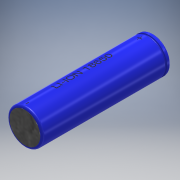
# Autodesk Inventor part: Bateria 18650
Saved by Autodesk Inventor 2018 (Build 220112000, 112)
## iProperties
Created: 2017-09-13
Part Number: Bateria 18650
Material: Genérico
Document SubType Name: Modeling
Designer: Julio Orozco
Density: 1 g/cm^3
Appearance: Valor por defecto
Author: Julio Orozco
Autodesk Inventor part; units mm, degrees
note: some values were not read from the file. Chosen so that the rebuilt part matches the saved one: direction of "Repujado1".
ref_plane "YZ Plane" through (0, 0, 0) normal (1, 0, 0) x (0, 1, 0)
sketch "Boceto1" plane through (0, 0, 0) normal (0, 1, 0) x (-1, 0, 0)
  circle A0 centre (0, 0) radius 9
  dimension "d0" = 18
  constraints: 1 centre point, 1 coincident
  measures "d0" diameter of A0
extrude "Extrusión1" add sketch "Boceto1" along normal blind 65
sketch "Boceto2" plane through (0, 0, 0) normal (0, 0, 1) x (1, 0, 0)
  line L0 (0, 0) -> (0, 65) construction
  line L1 (9, 65) -> (-9, 65) projected
  line L2 (9, 0) -> (9, 65) projected
  circle A0 centre (9, 62.5) radius 0.5
  dimension "d3" = 1
  dimension "d4" = 2.5
  constraints: 2 end point, 1 centre point, 1 midpoint, 1 point on line
  measures "d3" diameter of A0
  measures "d4" distance from line of A0.centre L1
revolve "Revolución1" cut sketch "Boceto2" angle 360 about axis through (0, 0, 0) along (0, 1, 0)
fillet "Empalme1" radius 1 2 edges at (9, 65, 0) (9, 0, 0)
ref_plane "Plano de trabajo1" through (0, 66, 0) normal (0, 1, 0) x (1, 0, 0)
sketch "Boceto3" plane through (0, 66, 0) normal (0, 1, 0) x (1, 0, 0)
  circle A0 centre (0, 0) radius 3.5
  dimension "d8" = 7
  constraints: 1 centre point, 1 coincident
  measures "d8" diameter of A0
extrude "Extrusión2" add sketch "Boceto3" against normal blind 0.1
sketch "Boceto4" plane through (0, 0, 0) normal (0, 0, 1) x (1, 0, 0)
  line L0 (-8, 65) -> (8, 65) projected
  line L1 (-3.5, 66) -> (3.5, 66) projected
  arc A0 (8, 65) -> (3.5, 66) centre (3.5, 55.375) ccw
  arc A1 (7.7585, 65) -> (3.5, 65.9) centre (3.5, 55.375) ccw
  line L2 (-3.5, 65.9) -> (3.5, 65.9) projected
  line L3 (3.5, 65.9) -> (3.5, 66)
  line L4 (7.7585, 65) -> (8, 65)
  line L5 (0, 65.9) -> (0, 63.9288) construction
  point P0 (0, 0)
  dimension "d11" = 0.1
  constraints: 6 end point, 4 point on circle, 2 centre point, 1 collinear, 1 midpoint, 1 perpendicular, 1 point on line, 1 tangent, 1 vertical
  measures "d11" radial gap between concentric circles of A0 A1
revolve "Revolución2" add sketch "Boceto4" angle 360 about axis through (0, 65.9, 0) along (0, -1, 0)
sketch "Boceto5" plane through (0, 66, 0) normal (0, 1, 0) x (1, 0, 0)
  line L0 (-6.8, -1.2007) -> (-6.8, 1.2993) construction
  line L1 (-5.6, -1.2007) -> (-5.6, 1.2993)
  line L2 (-8, 1.2993) -> (-8, -1.2007)
  arc A0 (-8, -1.2007) -> (-5.6, -1.2007) centre (-6.8, -1.2007) ccw
  arc A1 (-5.6, 1.2993) -> (-8, 1.2993) centre (-6.8, 1.2993) ccw
  point P0 (0, 0)
  point P1 (-6.8, 0.0493)
  dimension "d13" = 1.2
  dimension "d14" = 2.5
  dimension "d15" = 6.8
  constraints: 8 end point, 4 point on circle, 4 tangent, 2 centre point, 1 midpoint, 1 parallel, 1 vertical
  measures "d13" radius of A1
  measures "d14" distance of L1.start L1.end
  measures "d15" horizontal distance of point (0, 0) point (-6.8, 0.049)
extrude "Extrusión4" cut sketch "Boceto5" against normal blind 1
pattern_circular "Patrón circular1" count 6 over 360 about axis through (0, 0, 0) along (0, 1, 0) of "Extrusión4"
sketch "Boceto6" plane through (0, 0, 0) normal (0, -1, 0) x (1, 0, 0)
  circle A0 centre (0, 0) radius 7.7585
  constraints: 1 centre point, 1 coincident
extrude "Extrusión5" add sketch "Boceto6" along normal blind 0.1
ref_plane "Plano de trabajo2" through (0, 0, 9) normal (0, 0, 1) x (1, 0, 0)
sketch "Boceto7" plane through (0, 0, 9) normal (0, 0, 1) x (1, 0, 0)
  line L0 (-3.1701, 1.4356) -> (-3.1701, 76.7108) construction
  line L1 (-3.1701, 76.7108) -> (-0.0107, 76.7108) construction
  line L2 (-0.0107, 76.7108) -> (-0.0107, 1.4356) construction
  line L3 (-0.0107, 1.4356) -> (-3.1701, 1.4356) construction
  line L4 (-1.0179, 1.6337) -> (-1.3827, 1.6337)
  line L5 (-1.3827, 1.6337) -> (-1.3827, 3.1602)
  line L6 (-1.3827, 3.1602) -> (-1.0179, 3.1602)
  line L7 (-1.0179, 3.1602) -> (-1.0179, 1.6337)
  line L8 (-0.0904, 16.1602) -> (-3.0904, 16.1602)
  line L9 (-3.0904, 16.1602) -> (-3.0904, 16.5853)
  line L10 (-3.0904, 16.5853) -> (-0.4938, 16.5853)
  line L11 (-0.4938, 16.5853) -> (-0.4938, 18.4211)
  line L12 (-0.4938, 18.4211) -> (-0.0904, 18.4211)
  line L13 (-0.0904, 18.4211) -> (-0.0904, 16.1602)
  line L14 (-0.0904, 18.8535) -> (-3.0904, 18.8535)
  line L15 (-3.0904, 18.8535) -> (-3.0904, 19.2786)
  line L16 (-3.0904, 19.2786) -> (-0.0904, 19.2786)
  line L17 (-0.0904, 19.2786) -> (-0.0904, 18.8535)
  line L18 (-1.0179, 19.8486) -> (-1.3827, 19.8486)
  line L19 (-1.3827, 19.8486) -> (-1.3827, 21.3752)
  line L20 (-1.3827, 21.3752) -> (-1.0179, 21.3752)
  line L21 (-1.0179, 21.3752) -> (-1.0179, 19.8486)
  line L22 (-0.0904, 21.9477) -> (-3.0904, 21.9477)
  line L23 (-3.0904, 21.9477) -> (-3.0904, 22.3728)
  line L24 (-3.0904, 22.3728) -> (-0.0904, 22.3728)
  line L25 (-0.0904, 22.3728) -> (-0.0904, 21.9477)
  spline S0 degree 2 poles (-1.5904, 22.9235) (-2.315, 22.9235) (-3.1701, 23.81) (-3.1701, 24.5684) knots 0 0 0 1 2 2 2
  spline S1 degree 2 poles (-3.1701, 24.5684) (-3.1701, 25.3269) (-2.315, 26.211) (-1.5904, 26.211) knots 0 0 0 1 2 2 2
  spline S2 degree 2 poles (-1.5904, 26.211) (-0.8634, 26.211) (-0.0107, 25.3245) (-0.0107, 24.566) knots 0 0 0 1 2 2 2
  spline S3 degree 2 poles (-0.0107, 24.566) (-0.0107, 23.8076) (-0.8634, 22.9235) (-1.5904, 22.9235) knots 0 0 0 1 2 2 2
  spline S4 degree 2 poles (-1.5904, 23.3631) (-1.0324, 23.3631) (-0.4093, 24.0008) (-0.4093, 24.5684) knots 0 0 0 1 2 2 2
  spline S5 degree 2 poles (-0.4093, 24.5684) (-0.4093, 25.1361) (-1.0349, 25.7713) (-1.5904, 25.7713) knots 0 0 0 1 2 2 2
  spline S6 degree 2 poles (-1.5904, 25.7713) (-2.146, 25.7713) (-2.7716, 25.1337) (-2.7716, 24.566) knots 0 0 0 1 2 2 2
  spline S7 degree 2 poles (-2.7716, 24.566) (-2.7716, 23.9984) (-2.146, 23.3631) (-1.5904, 23.3631) knots 0 0 0 1 2 2 2
  line L26 (-0.0904, 26.7327) -> (-3.0904, 26.7327)
  line L27 (-3.0904, 26.7327) -> (-3.0904, 27.3076)
  line L28 (-3.0904, 27.3076) -> (-0.53, 29.1965)
  line L29 (-0.53, 29.1965) -> (-3.0904, 29.1965)
  line L30 (-3.0904, 29.1965) -> (-3.0904, 29.6071)
  line L31 (-3.0904, 29.6071) -> (-0.0904, 29.6071)
  line L32 (-0.0904, 29.6071) -> (-0.0904, 29.0346)
  line L33 (-0.0904, 29.0346) -> (-2.6508, 27.1481)
  line L34 (-2.6508, 27.1481) -> (-0.0904, 27.1481)
  line L35 (-0.0904, 27.1481) -> (-0.0904, 26.7327)
  line L36 (-0.0904, 32.6385) -> (-2.1991, 32.6385)
  line L37 (-2.1991, 32.6385) -> (-2.1991, 31.7448)
  line L38 (-2.1991, 31.7448) -> (-2.5445, 31.7448)
  line L39 (-2.5445, 31.7448) -> (-2.5445, 31.81)
  spline S8 degree 2 poles (-2.5445, 31.81) (-2.5445, 32.2617) (-2.8054, 32.7013) (-3.0904, 32.7303) knots 0 0 0 1 2 2 2
  line L40 (-3.0904, 32.7303) -> (-3.0904, 33.0467)
  line L41 (-3.0904, 33.0467) -> (-0.0904, 33.0467)
  line L42 (-0.0904, 33.0467) -> (-0.0904, 32.6385)
  spline S9 degree 2 poles (-1.6991, 34.9573) (-1.7643, 34.694) (-2.0759, 34.4163) (-2.3006, 34.4163) knots 0 0 0 1 2 2 2
  spline S10 degree 2 poles (-2.3006, 34.4163) (-2.6653, 34.4163) (-3.0904, 35.0081) (-3.0904, 35.525) knots 0 0 0 1 2 2 2
  spline S11 degree 2 poles (-3.0904, 35.525) (-3.0904, 36.0032) (-2.658, 36.5781) (-2.3006, 36.5781) knots 0 0 0 1 2 2 2
  spline S12 degree 2 poles (-2.3006, 36.5781) (-2.0759, 36.5781) (-1.7643, 36.2979) (-1.6991, 36.037) knots 0 0 0 1 2 2 2
  spline S13 degree 2 poles (-1.6991, 36.037) (-1.6291, 36.3655) (-1.2474, 36.694) (-0.9382, 36.694) knots 0 0 0 1 2 2 2
  spline S14 degree 2 poles (-0.9382, 36.694) (-0.5059, 36.694) (-0.0107, 36.0564) (-0.0107, 35.496) knots 0 0 0 1 2 2 2
  spline S15 degree 2 poles (-0.0107, 35.496) (-0.0107, 34.9404) (-0.5107, 34.2955) (-0.9382, 34.2955) knots 0 0 0 1 2 2 2
  spline S16 degree 2 poles (-0.9382, 34.2955) (-1.245, 34.2955) (-1.6411, 34.6385) (-1.6991, 34.9573) knots 0 0 0 1 2 2 2
  spline S17 degree 2 poles (-0.9745, 36.2544) (-1.2281, 36.2544) (-1.5131, 35.851) (-1.5131, 35.4887) knots 0 0 0 1 2 2 2
  spline S18 degree 2 poles (-1.5131, 35.4887) (-1.5131, 35.1216) (-1.2305, 34.7206) (-0.9745, 34.7206) knots 0 0 0 1 2 2 2
  spline S19 degree 2 poles (-0.9745, 34.7206) (-0.7112, 34.7206) (-0.402, 35.1288) (-0.402, 35.4767) knots 0 0 0 1 2 2 2
  spline S20 degree 2 poles (-0.402, 35.4767) (-0.402, 35.8438) (-0.7039, 36.2544) (-0.9745, 36.2544) knots 0 0 0 1 2 2 2
  spline S21 degree 2 poles (-2.3006, 36.1361) (-2.5059, 36.1361) (-2.7329, 35.8076) (-2.7329, 35.5081) knots 0 0 0 1 2 2 2
  spline S22 degree 2 poles (-2.7329, 35.5081) (-2.7329, 35.1892) (-2.5107, 34.8535) (-2.3006, 34.8535) knots 0 0 0 1 2 2 2
  spline S23 degree 2 poles (-2.3006, 34.8535) (-2.0928, 34.8535) (-1.8465, 35.1989) (-1.8465, 35.496) knots 0 0 0 1 2 2 2
  spline S24 degree 2 poles (-1.8465, 35.496) (-1.8465, 35.7931) (-2.0928, 36.1361) (-2.3006, 36.1361) knots 0 0 0 1 2 2 2
  spline S25 degree 2 poles (-1.5735, 37.496) (-1.8054, 37.6699) (-2.03, 38.1482) (-2.03, 38.4549) knots 0 0 0 1 2 2 2
  spline S26 degree 2 poles (-2.03, 38.4549) (-2.03, 38.9283) (-1.4938, 39.5105) (-1.0614, 39.5105) knots 0 0 0 1 2 2 2
  spline S27 degree 2 poles (-1.0614, 39.5105) (-0.5952, 39.5105) (-0.0107, 38.8317) (-0.0107, 38.2858) knots 0 0 0 1 2 2 2
  spline S28 degree 2 poles (-0.0107, 38.2858) (-0.0107, 37.6892) (-0.7667, 37.0467) (-1.4696, 37.0467) knots 0 0 0 1 2 2 2
  spline S29 degree 2 poles (-1.4696, 37.0467) (-2.2522, 37.0467) (-3.0952, 37.7254) (-3.0952, 38.3559) knots 0 0 0 1 2 2 2
  spline S30 degree 2 poles (-3.0952, 38.3559) (-3.0952, 38.7834) (-2.7088, 39.3196) (-2.3585, 39.3776) knots 0 0 0 1 2 2 2
  line L43 (-2.3585, 39.3776) -> (-2.3585, 38.9525)
  spline S31 degree 2 poles (-2.3585, 38.9525) (-2.5421, 38.8945) (-2.7329, 38.5902) (-2.7329, 38.3559) knots 0 0 0 1 2 2 2
  spline S32 degree 2 poles (-2.7329, 38.3559) (-2.7329, 37.9259) (-2.1532, 37.496) (-1.5735, 37.496) knots 0 0 0 1 2 2 2
  spline S33 degree 2 poles (-1.0276, 37.5515) (-0.7498, 37.5515) (-0.4093, 37.9597) (-0.4093, 38.2931) knots 0 0 0 1 2 2 2
  spline S34 degree 2 poles (-0.4093, 38.2931) (-0.4093, 38.653) (-0.7547, 39.0829) (-1.0373, 39.0829) knots 0 0 0 1 2 2 2
  spline S35 degree 2 poles (-1.0373, 39.0829) (-1.3223, 39.0829) (-1.6725, 38.6602) (-1.6725, 38.3148) knots 0 0 0 1 2 2 2
  spline S36 degree 2 poles (-1.6725, 38.3148) (-1.6725, 37.9791) (-1.3102, 37.5515) (-1.0276, 37.5515) knots 0 0 0 1 2 2 2
  line L44 (-0.8948, 39.8414) -> (-0.8948, 40.2689)
  spline S37 degree 2 poles (-0.8948, 40.2689) (-0.6484, 40.31) (-0.3972, 40.6651) (-0.3972, 40.9718) knots 0 0 0 1 2 2 2
  spline S38 degree 2 poles (-0.3972, 40.9718) (-0.3972, 41.3269) (-0.7716, 41.7641) (-1.0687, 41.7641) knots 0 0 0 1 2 2 2
  spline S39 degree 2 poles (-1.0687, 41.7641) (-1.3634, 41.7641) (-1.7281, 41.3366) (-1.7281, 40.9936) knots 0 0 0 1 2 2 2
  spline S40 degree 2 poles (-1.7281, 40.9936) (-1.7281, 40.7689) (-1.5687, 40.4332) (-1.4117, 40.3366) knots 0 0 0 1 2 2 2
  line L45 (-1.4117, 40.3366) -> (-1.4117, 39.9211)
  line L46 (-1.4117, 39.9211) -> (-3.0155, 40.182)
  line L47 (-3.0155, 40.182) -> (-3.0155, 41.9815)
  line L48 (-3.0155, 41.9815) -> (-2.6363, 41.9815)
  line L49 (-2.6363, 41.9815) -> (-2.6363, 40.5032)
  line L50 (-2.6363, 40.5032) -> (-1.8102, 40.3607)
  spline S41 degree 2 poles (-1.8102, 40.3607) (-1.9431, 40.4936) (-2.0759, 40.868) (-2.0759, 41.1095) knots 0 0 0 1 2 2 2
  spline S42 degree 2 poles (-2.0759, 41.1095) (-2.0759, 41.3003) (-1.989, 41.6312) (-1.902, 41.7641) knots 0 0 0 1 2 2 2
  spline S43 degree 2 poles (-1.902, 41.7641) (-1.7667, 41.9718) (-1.3465, 42.2061) (-1.1001, 42.2061) knots 0 0 0 1 2 2 2
  spline S44 degree 2 poles (-1.1001, 42.2061) (-0.6146, 42.2061) (-0.0107, 41.5274) (-0.0107, 40.9742) knots 0 0 0 1 2 2 2
  spline S45 degree 2 poles (-0.0107, 40.9742) (-0.0107, 40.4887) (-0.4793, 39.8873) (-0.8948, 39.8414) knots 0 0 0 1 2 2 2
  spline S46 degree 2 poles (-1.5518, 42.6047) (-2.2909, 42.6047) (-3.0904, 43.2279) (-3.0904, 43.8052) knots 0 0 0 1 2 2 2
  spline S47 degree 2 poles (-3.0904, 43.8052) (-3.0904, 44.3849) (-2.2933, 45.0105) (-1.5518, 45.0105) knots 0 0 0 1 2 2 2
  spline S48 degree 2 poles (-1.5518, 45.0105) (-0.8102, 45.0105) (-0.0107, 44.3849) (-0.0107, 43.8052) knots 0 0 0 1 2 2 2
  spline S49 degree 2 poles (-0.0107, 43.8052) (-0.0107, 43.2303) (-0.8126, 42.6047) (-1.5518, 42.6047) knots 0 0 0 1 2 2 2
  spline S50 degree 2 poles (-1.5518, 43.037) (-0.9721, 43.037) (-0.3972, 43.4211) (-0.3972, 43.81) knots 0 0 0 1 2 2 2
  spline S51 degree 2 poles (-0.3972, 43.81) (-0.3972, 44.1989) (-0.9672, 44.5781) (-1.5518, 44.5781) knots 0 0 0 1 2 2 2
  spline S52 degree 2 poles (-1.5518, 44.5781) (-2.1363, 44.5781) (-2.7064, 44.1989) (-2.7064, 43.81) knots 0 0 0 1 2 2 2
  spline S53 degree 2 poles (-2.7064, 43.81) (-2.7064, 43.4211) (-2.1315, 43.037) (-1.5518, 43.037) knots 0 0 0 1 2 2 2
  line L51 (-2.5663, 59.5225) -> (-1.4696, 59.5225)
  line L52 (-1.4696, 59.5225) -> (-1.4696, 60.5926)
  line L53 (-1.4696, 60.5926) -> (-1.187, 60.5926)
  line L54 (-1.187, 60.5926) -> (-1.187, 59.5225)
  line L55 (-1.187, 59.5225) -> (-0.0904, 59.5225)
  line L56 (-0.0904, 59.5225) -> (-0.0904, 59.2351)
  line L57 (-0.0904, 59.2351) -> (-1.187, 59.2351)
  line L58 (-1.187, 59.2351) -> (-1.187, 58.1651)
  line L59 (-1.187, 58.1651) -> (-1.4696, 58.1651)
  line L60 (-1.4696, 58.1651) -> (-1.4696, 59.2351)
  line L61 (-1.4696, 59.2351) -> (-2.5663, 59.2351)
  line L62 (-2.5663, 59.2351) -> (-2.5663, 59.5225)
  point P0 (0, 0)
  constraints: 2 other
emboss "Repujado1" sketch "Boceto7" operation cut depth 0.1 direction (0, 0, -1)
